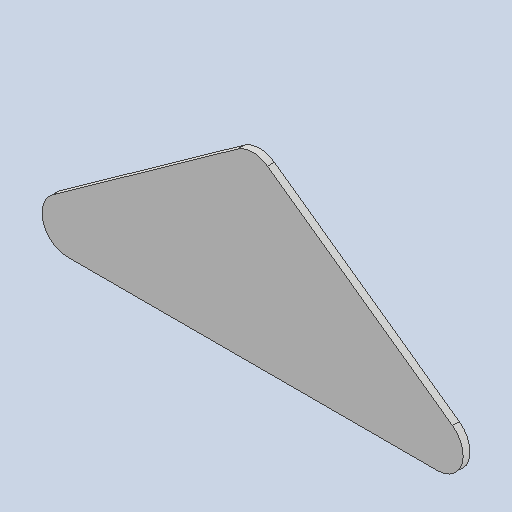
# Autodesk Inventor part: NDV-3003 Branch roof cap 01
Saved by Autodesk Inventor 2026.2 (Build 302298000, 298)
## iProperties
Created: 2026-10-05
Part Number: NDV-3003 Branch roof cap 01
Material: Generic
Document SubType Name: Sheet Metal
Designer: admin
Density: 1 g/cm^3
Sheet Metal Rule: Default_mm
Appearance: Default
Stock Number: Заглушка домика
Author: admin
Autodesk Inventor part; units mm, degrees
ref_plane "YZ Plane" through (0, 0, 0) normal (1, 0, 0) x (0, 1, 0)
ref_plane "XZ Plane" through (0, 0, 0) normal (0, 1, 0) x (-1, 0, 0)
ref_plane "XY Plane" through (0, 0, 0) normal (0, 0, 1) x (1, 0, 0)
derived "NDV-0010 Parameters 01.ipt"
sketch "sk_cap" plane through (0, 0, 0) normal (0, 0, 1) x (1, 0, 0)
  line L0 (-31, 0) -> (31, 0)
  line L1 (31, 0) -> (0, 22.1429)
  line L2 (0, 22.1429) -> (-31, 0)
  point P0 (0, 0)
  dimension "d5" = 62
  dimension "d6" = 22.1429
  measures "d5" distance of L0.start L0.end
  measures "d6" vertical distance of L0.start L1.end
extrude "Plate2" add sketch "sk_cap" along normal blind 0.8
fillet "Corner Round1" radius 3 3 edges at (0, 22.1429, 0.4) (-31, 0, 0.4) (31, 0, 0.4)
equation "\"d5\" = Roof_cap_w"
equation "\"d6\" = Roof_cap_h"
equation "\"d8\" = Roof_cap_R"
equation "\"d7\" = Thickness"
equation "\"Thickness\" = Roof_cap_t"
equation "\"BendRadius\" = Thickness"
equation "\"BendReliefWidth\" = Thickness"
equation "\"BendReliefDepth\" = 0.5 * Thickness"
equation "\"CornerReliefSize\" = 4 * Thickness"
equation "\"MinimumRemnant\" = 2 * Thickness"
equation "\"TransitionRadius\" = BendRadius"
equation "\"JacobiRadiusSize\" = BendRadius"
equation "\"GapSize\" = Thickness"
equation "\"Roof_cap_w\" = 62"
equation "\"Roof_cap_h\" = 22.142857"
equation "\"Roof_cap_R\" = 3"
equation "\"Roof_cap_t\" = 0.8"
body "Solid2"
